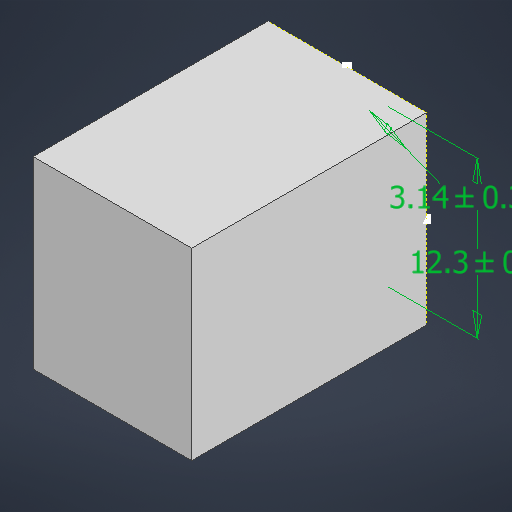
# Autodesk Inventor part: Adafruit_1528-4663-ND
Saved by Autodesk Inventor 2026.2 (Build 302298000, 298)
## iProperties
Created: 2026-01-28
Part Number: Adafruit_1528-4663-ND
Material: Generic
Document SubType Name: Modeling
Designer: vckot
Density: 1 g/cm^3
Appearance: Default
Author: vckot
Autodesk Inventor part; units mm, degrees
ref_plane "YZ Plane" through (0, 0, 0) normal (1, 0, 0) x (0, 1, 0)
ref_plane "XZ Plane" through (0, 0, 0) normal (0, 1, 0) x (-1, 0, 0)
ref_plane "XY Plane" through (0, 0, 0) normal (0, 0, 1) x (1, 0, 0)
sketch "Sketch1" plane through (0, 0, 0) normal (0, 0, 1) x (1, 0, 0)
  line L0 (0, 0) -> (12.5, 0)
  line L1 (12.5, 0) -> (12.5, 14.5)
  line L2 (12.5, 14.5) -> (0, 14.5)
  line L3 (0, 14.5) -> (0, 0)
  dimension "d0" = 14.5
  dimension "d1" = 12.5
  constraints: 8 end point, 2 parallel, 1 horizontal, 1 perpendicular
  measures "d0" distance of L0.end L1.end
  measures "d1" distance of L1.end L2.end
extrude "Extrusion1" add sketch "Sketch1" against normal blind 18.5
sketch "Sketch2" plane through (0, 0, -18.5) normal (0, 0, -1) x (-1, 0, 0)
  circle A0 centre (-9.4446, 2.67) radius 1.57
  circle A1 centre (-3.0554, 2.67) radius 1.57
  circle A2 centre (-3.0554, 11.83) radius 1.57
  circle A3 centre (-9.4446, 11.83) radius 1.57
  line L0 (-9.4446, 11.83) -> (-9.4446, 2.67) construction
  line L1 (-12.5, 14.5) -> (-12.5, 0) construction
  line L2 (-9.4446, 11.83) -> (-3.0554, 11.83) construction
  line L3 (0, 14.5) -> (-12.5, 14.5) construction
  point P0 (0, 0)
  point P1 (-9.4446, 7.25)
  point P2 (-12.5, 7.25)
  point P3 (-6.25, 11.83)
  point P4 (-6.25, 14.5)
  dimension "d4" = 3.14
  dimension "d5" = 12.3
  constraints: 4 centre point, 4 end point, 4 midpoint, 3 equal radius, 3 horizontal alignment, 3 vertical alignment, 1 horizontal, 1 vertical
  measures "d4" diameter of A3
body "Solid1"
